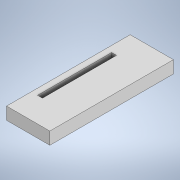
# Autodesk Inventor part: floor_side
Saved by Autodesk Inventor 2021 (Build 250183000, 183)
## iProperties
Created: 2020-06-13
Part Number: floor_side
Material: Generic
Document SubType Name: Modeling
Designer: Yatekii
Density: 1 g/cm^3
Appearance: Default
Author: Yatekii
Autodesk Inventor part; units mm, degrees
ref_plane "YZ Plane" through (0, 0, 0) normal (1, 0, 0) x (0, 1, 0)
ref_plane "XZ Plane" through (0, 0, 0) normal (0, 1, 0) x (-1, 0, 0)
ref_plane "XY Plane" through (0, 0, 0) normal (0, 0, 1) x (1, 0, 0)
sketch "Sketch1" plane through (0, 0, 0) normal (0, 1, 0) x (-1, 0, 0)
  line L0 (-17.5, -50) -> (17.5, -50)
  line L1 (17.5, -50) -> (17.5, 50)
  line L2 (17.5, 50) -> (-17.5, 50)
  line L3 (-17.5, 50) -> (-17.5, -50)
  line L4 (-17.5, -50) -> (17.5, 50) construction
  line L5 (17.5, -50) -> (-17.5, 50) construction
  point P0 (0, 0)
  dimension "d0" = 35
  dimension "d1" = 100
  constraints: 12 end point, 2 midpoint, 2 parallel, 1 horizontal, 1 perpendicular
  measures "d0" distance of L2.end L1.end
  measures "d1" distance of L1.end L0.end
extrude "Extrusion1" add sketch "Sketch1" along normal blind 10
sketch "Sketch2" plane through (0, 10, 0) normal (0, 1, 0) x (1, 0, 0)
  line L0 (-8.5, 30) -> (-12.5, 30)
  line L1 (-12.5, 30) -> (-12.5, -30)
  line L2 (-12.5, -30) -> (-8.5, -30)
  line L3 (-8.5, -30) -> (-8.5, 30)
  line L4 (-8.5, 30) -> (-12.5, -30) construction
  line L5 (-12.5, 30) -> (-8.5, -30) construction
  line L6 (-17.5, 50) -> (-17.5, -50) projected
  point P0 (0, 0)
  point P1 (-10.5, 0)
  dimension "d4" = 4
  dimension "d5" = 60
  dimension "d9" = 5
  constraints: 12 end point, 2 midpoint, 2 parallel, 1 horizontal, 1 perpendicular
  measures "d4" distance of L2.end L1.end
  measures "d5" distance of L1.end L0.end
  measures "d9" distance between parallel lines of L6 L1
extrude "Extrusion2" cut sketch "Sketch2" against normal blind 10
body "Solid1"
